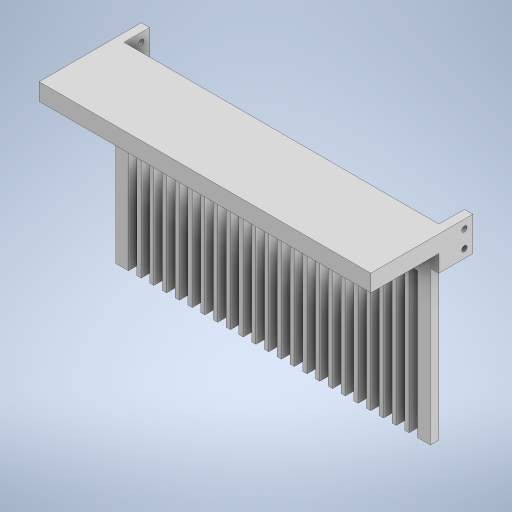
# Autodesk Inventor part: 猫铲
Saved by Autodesk Inventor 2023.1 (Build 271208000, 208)
## iProperties
Created: 2023-07-14
Part Number: 猫铲
Material: 常规
Document SubType Name: Modeling
Designer: Selcon
Density: 1 g/cm^3
Appearance: 默认
Author: Selcon
Autodesk Inventor part; units mm, degrees
ref_plane "YZ Plane" through (0, 0, 0) normal (1, 0, 0) x (0, 1, 0)
ref_plane "XZ Plane" through (0, 0, 0) normal (0, 1, 0) x (-1, 0, 0)
ref_plane "XY Plane" through (0, 0, 0) normal (0, 0, 1) x (1, 0, 0)
sketch "草图1" plane through (0, 0, 0) normal (0, 0, 1) x (1, 0, 0)
  line L0 (-185, 220) -> (185, 220)
  line L1 (185, 220) -> (185, 0)
  line L2 (185, 0) -> (-185, 0)
  line L3 (-185, 0) -> (-185, 220)
  line L4 (0, -44) -> (0, 264) projected
  line L5 (-259, 0) -> (259, 0) projected
  point P0 (0, 0)
  point P1 (0, 0)
  dimension "d0" = 370
  dimension "d1" = 220
  constraints: 8 end point, 2 midpoint, 2 parallel, 1 horizontal, 1 perpendicular, 1 other
  measures "d0" distance of L0.start L0.end
  measures "d1" distance of L0.end L1.end
extrude "拉伸1" add sketch "草图1" along normal blind 10
sketch "草图2" plane through (0, 0, 10) normal (0, 0, 1) x (1, 0, 0)
  line L0 (-170, 170) -> (-160, 170)
  line L1 (-160, 170) -> (-160, 0)
  line L2 (-160, 0) -> (-170, 0)
  line L3 (-170, 0) -> (-170, 170)
  line L4 (-185, 220) -> (-185, 0) projected
  line L5 (185, 220) -> (-185, 220) projected
  point P0 (0, 0)
  point P1 (-165, 170)
  dimension "d5" = 15
  dimension "d6" = 10
  dimension "d7" = 50
  constraints: 8 end point, 2 parallel, 1 horizontal, 1 midpoint, 1 perpendicular
  measures "d5" distance between parallel lines of L3 L4
  measures "d6" distance of L1.end L2.end
  measures "d7" distance from line of L5 point (-165, 170)
extrude "拉伸2" cut sketch "草图2" against normal through all
pattern_linear "矩形阵列1" count 23 spacing 15 along (1, 0, 0) of "拉伸2"
sketch "草图3" plane through (185, 0, 0) normal (1, 0, 0) x (0, 0, -1)
  line L0 (-10, 0) -> (-10, 220) projected
  line L1 (-10, 220) -> (30, 220)
  line L2 (30, 220) -> (30, 180)
  line L3 (30, 180) -> (-10, 180)
  line L4 (-10, 180) -> (-10, 220)
  point P0 (0, 0)
  point P1 (-10, 180)
  dimension "d13" = 40
  dimension "d14" = 40
  constraints: 8 end point, 2 parallel, 1 horizontal, 1 perpendicular
  measures "d13" distance of L1.end L2.end
  measures "d14" distance of L2.end L3.end
extrude "拉伸3" add sketch "草图3" along normal blind 10
sketch "草图5" plane through (195, 0, 0) normal (1, 0, 0) x (0, 0, -1)
  line L0 (0, 180) -> (0, 220) projected
  line L1 (-10, 180) -> (30, 180) projected
  point P0 (0, 0)
  point P1 (20, 210)
  point P2 (20, 190)
  dimension "d35" = 20
  dimension "d36" = 20
  dimension "d37" = 10
  constraints: 1 vertical alignment
  measures "d35" distance of point (20, 190) point (20, 210)
  measures "d36" distance from line of L0 point (20, 190)
  measures "d37" distance from line of L1 point (20, 190)
hole "孔2" at (195, 210, -20) at (195, 190, -20) direction (-1, 0, 0) diameter 6.4008 end through all thread size "5/16-18 UNC" class "2B" standard "ANSI Unified Screw Threads"
mirror "镜像2" about plane through (0, 0, 0) normal (1, 0, 0) of "拉伸3", "孔2"
sketch "草图6" plane through (0, 0, 10) normal (0, 0, 1) x (1, 0, 0)
  line L0 (-195, 220) -> (195, 220) projected
  line L1 (195, 220) -> (195, 180) projected
  line L2 (-195, 220) -> (195, 220)
  line L3 (195, 220) -> (195, 200)
  line L4 (195, 200) -> (-195, 200)
  line L5 (-195, 200) -> (-195, 220)
  point P0 (0, 0)
  constraints: 8 end point, 2 parallel, 1 horizontal, 1 midpoint, 1 perpendicular
extrude "拉伸4" add sketch "草图6" along normal blind 80
